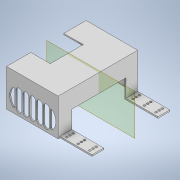
# Autodesk Inventor part: Enclosure
Saved by Autodesk Inventor 2020 (Build 240168000, 168)
## iProperties
Created: 2020-02-08
Part Number: Enclosure
Material: Generic
Document SubType Name: Modeling
Designer: pp445
Density: 1 g/cm^3
Appearance: Default
Author: pp445
Autodesk Inventor part; units mm, degrees
ref_plane "YZ Plane" through (0, 0, 0) normal (1, 0, 0) x (0, 1, 0)
ref_plane "XZ Plane" through (0, 0, 0) normal (0, 1, 0) x (-1, 0, 0)
ref_plane "XY Plane" through (0, 0, 0) normal (0, 0, 1) x (1, 0, 0)
sketch "Sketch1" plane through (0, 0, 0) normal (0, 1, 0) x (-1, 0, 0)
  line L0 (0, 0) -> (81, 0)
  line L1 (81, 0) -> (81, -120)
  line L2 (81, -120) -> (0, -120)
  line L3 (0, -120) -> (0, 0)
  line L4 (217, 30) -> (81, 30)
  line L5 (81, 30) -> (81, -146)
  line L6 (81, -146) -> (217, -146)
  line L7 (217, -146) -> (217, 30)
  line L8 (81, -60) -> (0, -60) construction
  dimension "d0" = 120
  dimension "d1" = 81
  dimension "d2" = 176
  dimension "d4" = 136
  dimension "d40" = 26
  constraints: 18 end point, 4 parallel, 2 horizontal, 2 perpendicular, 1 collinear, 1 midpoint, 1 point on line
  measures "d0" distance of L2.end L0.start
  measures "d1" distance of L0.start L0.end
  measures "d2" distance between parallel lines of L6 L4
  measures "d4" distance of L4.start L4.end
  measures "d40" distance between parallel lines of L2 L6
extrude "Extrusion1" add sketch "Sketch1" against normal blind 82
shell "Shell1" thickness 2.54 removed faces 3 at (-171.6667, -82, -38.6667) at (0, -54.6667, -40) at (-217, -27.3333, -87.3333)
sketch "Sketch3" plane through (0, -82, 0) normal (0, -1, 0) x (1, 0, 0)
  line L0 (-81, -146) -> (-81, -120) projected
  line L1 (0, -2.54) -> (0, 0) projected
  line L2 (0, 0) -> (-81, 0)
  line L3 (-81, -120) -> (0, -120) projected
  line L4 (0, -120) -> (-81, -120)
  line L5 (-81, -120) -> (-81, -146)
  line L6 (-81, -146) -> (0, -146)
  line L7 (0, -146) -> (0, -120)
  line L8 (-81, 0) -> (-81, 30) projected
  line L9 (-81, 0) -> (0, 0) projected
  line L10 (-217, 30) -> (-81, 30) projected
  line L11 (0, 0) -> (-81, 0)
  line L12 (-81, 0) -> (-81, 30)
  line L13 (-81, 30) -> (0, 30)
  line L14 (0, 30) -> (0, 0)
  constraints: 18 end point, 4 parallel, 3 horizontal, 2 perpendicular
extrude "Extrusion3" add sketch "Sketch3" against normal blind 3.175
sketch "Sketch5" plane through (0, -78.825, 0) normal (0, 1, 0) x (1, 0, 0)
  line L0 (0, 120) -> (0, 146) projected
  line L1 (0, 146) -> (-81, 146) projected
  line L2 (-81, 120) -> (-81, 146) projected
  line L3 (0, 120) -> (-81, 120) projected
  line L4 (-81, 0) -> (0, 0) projected
  line L5 (-81, -30) -> (-81, 0) projected
  line L6 (-81, -30) -> (0, -30) projected
  line L7 (0, -30) -> (0, 0) projected
  line L8 (0, 146) -> (0, 117.46) projected
  line L9 (-81, 120) -> (-81, 146) projected
  line L10 (0, 2.54) -> (0, -30) projected
  line L11 (0, -15) -> (-81, -15) construction
  line L12 (-81, -30) -> (-81, 0) projected
  circle A0 centre (-20.7, -15) radius 2.3813
  circle A1 centre (-46.1, -15) radius 2.3813
  circle A2 centre (-71.5, -15) radius 2.3813
  circle A3 centre (-20.7, 133.3) radius 2.3813
  circle A4 centre (-46.1, 133.3) radius 2.3813
  circle A5 centre (-71.5, 133.3) radius 2.3813
  line L13 (-81, 133.3) -> (0, 133.3) construction
  dimension "d18" = 20.7
  dimension "d19" = 25.4
  dimension "d20" = 25.4
  dimension "d21" = 4.7625
  dimension "d22" = 4.7625
  dimension "d23" = 4.7625
  dimension "d41" = 4.7625
  dimension "d42" = 4.7625
  dimension "d43" = 4.7625
  dimension "d44" = 20.7
  dimension "d45" = 25.4
  dimension "d46" = 25.4
  dimension "d47" = 13.3
  constraints: 9 point on line, 6 centre point, 4 end point, 1 midpoint, 1 perpendicular
  measures "d18" distance from line of L7 A0.centre
  measures "d19" distance of A0.centre A1.centre
  measures "d20" distance of A1.centre A2.centre
  measures "d21" diameter of A0
  measures "d22" diameter of A1
  measures "d23" diameter of A2
  measures "d41" diameter of A3
  measures "d42" diameter of A4
  measures "d43" diameter of A5
  measures "d44" distance from line of L8 A3.centre
  measures "d45" distance of A3.centre A4.centre
  measures "d46" distance of A4.centre A5.centre
  measures "d47" distance between parallel lines of L3 L13
extrude "Extrusion4" cut sketch "Sketch5" against normal up to surface (3.175 mm away) contours A3 | A4 | A5
ref_plane "Work Plane1" through (0, -2.54, -60) normal (0, 0, -1) x (-1, 0, 0)
mirror "Mirror1" about plane through (0, -2.54, -60) normal (0, 0, -1) of "Extrusion4"
sketch "Sketch6" plane through (0, 0, 0) normal (0, 1, 0) x (1, 0, 0)
  line L0 (-81, 120) -> (-81, 146) projected
  line L1 (-81, 146) -> (-217, 146) projected
  line L2 (-217, 146) -> (-217, -30) projected
  line L3 (-217, -30) -> (-81, -30) projected
  line L4 (-81, -30) -> (-81, 0) projected
  line L5 (-81, 0) -> (0, 0) projected
  line L6 (0, 0) -> (0, 120) projected
  line L7 (0, 120) -> (-81, 120) projected
  line L8 (-217, 143.46) -> (-217, -27.46) projected
  line L9 (-217, 60) -> (0, 60) construction
  line L10 (-217, 23.5) -> (-152, 23.5)
  line L11 (-152, 23.5) -> (-152, 96.5)
  line L12 (-152, 96.5) -> (-217, 96.5)
  line L13 (-217, 96.5) -> (-217, 23.5)
  line L14 (-217, 60) -> (-152, 60) construction
  dimension "d27" = 65
  constraints: 12 end point, 3 midpoint, 2 parallel, 2 point on line, 1 collinear, 1 horizontal, 1 perpendicular
  measures "d27" distance of L11.end L12.end
extrude "Extrusion5" cut sketch "Sketch6" against normal up to surface (2.54 mm away) contours L12 L11 L10 L2
sketch "Sketch7" plane through (-217, -82, -146) normal (-1, 0, 0) x (0, 0, 1)
  line L0 (0, 82) -> (49.5, 82) projected
  line L1 (49.5, 79.46) -> (49.5, 82) projected
  line L2 (0, 82) -> (49.5, 82) projected
  line L3 (0, 82) -> (0, 0) projected
  line L4 (2.54, 0) -> (0, 0) projected
  line L5 (2.54, 0) -> (2.54, 79.46) projected
  line L6 (2.54, 79.46) -> (49.5, 79.46) projected
  line L7 (122.5, 82) -> (122.5, 79.46) projected
  line L8 (122.5, 79.46) -> (173.46, 79.46) projected
  line L9 (173.46, 79.46) -> (173.46, 0) projected
  line L10 (176, 0) -> (173.46, 0) projected
  line L11 (176, 82) -> (176, 0) projected
  line L12 (122.5, 82) -> (176, 82) projected
  point P0 (146, 82)
  point P1 (49.5, 82)
extrude "Extrusion6" cut sketch "Sketch7" against normal blind 22
mirror "Mirror2" about plane through (0, -2.54, -60) normal (0, 0, -1) of "Extrusion4"
sketch "Sketch9" plane through (0, 0, 0) normal (1, 0, 0) x (0, 0, -1)
  line L0 (2.54, -82) -> (2.54, -2.54) projected
  line L1 (2.54, -2.54) -> (117.46, -2.54) projected
  line L2 (117.46, -2.54) -> (117.46, -82) projected
  line L3 (146, -82) -> (117.46, -82) projected
  line L4 (146, -82) -> (146, -78.825) projected
  line L5 (120, -78.825) -> (146, -78.825) projected
  line L6 (120, 0) -> (120, -78.825) projected
  line L7 (0, 0) -> (120, 0) projected
  line L8 (0, 0) -> (0, -78.825) projected
  line L9 (-30, -78.825) -> (0, -78.825) projected
  line L10 (-30, -82) -> (-30, -78.825) projected
  line L11 (2.54, -82) -> (-30, -82) projected
extrude "Extrusion8" cut sketch "Sketch9" against normal blind 10
sketch "Sketch10" plane through (-10, 0, 0) normal (1, 0, 0) x (0, 0, -1)
  line L0 (2.54, -82) -> (-30, -82) projected
  line L1 (2.54, -2.54) -> (2.54, -82) projected
  line L2 (117.46, -2.54) -> (2.54, -2.54) projected
  line L3 (117.46, -82) -> (117.46, -2.54) projected
  line L4 (146, -82) -> (117.46, -82) projected
  line L5 (146, -78.825) -> (146, -82) projected
  line L6 (120, -78.825) -> (146, -78.825) projected
  line L7 (120, 0) -> (120, -78.825) projected
  line L8 (0, 0) -> (120, 0) projected
  line L9 (0, -78.825) -> (0, 0) projected
  line L10 (-30, -78.825) -> (0, -78.825) projected
  line L11 (-30, -82) -> (-30, -78.825) projected
  line L12 (2.54, -82) -> (-30, -82) projected
  line L13 (-30, -78.825) -> (-26, -78.825)
  line L14 (-26, -78.825) -> (-26, -82)
  line L15 (-26, -82) -> (-30, -82)
  line L16 (-30, -82) -> (-30, -78.825)
  dimension "d50" = 4
  constraints: 8 end point, 2 parallel, 1 horizontal, 1 perpendicular, 1 point on line
  measures "d50" distance between parallel lines of L11 L14
extrude "Extrusion9" cut sketch "Sketch10" against normal up to surface (71 mm away) contours L0 L11 L10 L14
pattern_linear "Rectangular Pattern2" count 2 spacing 7 along (0, 0, -1) count 2 spacing 7 along (0, 0, 1) of "Extrusion4"
mirror "Mirror3" about plane through (0, -2.54, -60) normal (0, 0, -1) of "Extrusion4", "Rectangular Pattern2"
sketch "Sketch11" plane through (-81, -82, 30) normal (0, 0, 1) x (1, 0, 0)
  line L0 (0, 82) -> (0, 0) projected
  line L1 (-114, 82) -> (0, 82) projected
  line L2 (-114, 82) -> (-114, 0) projected
  line L3 (0, 0) -> (-114, 0) projected
  line L4 (-2.54, 0) -> (-114, 0) projected
  line L5 (-3.175, 0) -> (-109.175, 0)
  line L6 (-109.175, 0) -> (-109.175, 58.175)
  line L7 (-109.175, 58.175) -> (-3.175, 58.175)
  line L8 (-3.175, 58.175) -> (-3.175, 0)
  line L9 (-95.5478, 52.5) -> (-95.5478, 7.5)
  circle A0 centre (-79.7364, 30) radius 27.5 construction
  arc A1 (-95.5478, 52.5) -> (-95.5478, 7.5) centre (-79.7364, 30) ccw
  line L10 (-56.175, 58.175) -> (-56.175, 0) construction
  line L11 (-16.8022, 52.5) -> (-16.8022, 7.5)
  circle A2 centre (-32.6136, 30) radius 27.5 construction
  arc A3 (-16.8022, 7.5) -> (-16.8022, 52.5) centre (-32.6136, 30) ccw
  line L12 (-79.7364, 30) -> (-32.6136, 30) construction
  line L13 (-93.0078, 54) -> (-80.3078, 54)
  line L14 (-80.3078, 54) -> (-80.3078, 6)
  line L15 (-80.3078, 6) -> (-93.0078, 6)
  line L16 (-93.0078, 6) -> (-93.0078, 54)
  line L17 (-93.0078, 30) -> (-80.3078, 30) construction
  line L18 (-77.7678, 54) -> (-65.0678, 54)
  line L19 (-65.0678, 54) -> (-65.0678, 6)
  line L20 (-65.0678, 6) -> (-77.7678, 6)
  line L21 (-77.7678, 6) -> (-77.7678, 54)
  line L22 (-62.5278, 54) -> (-49.8278, 54)
  line L23 (-49.8278, 54) -> (-49.8278, 6)
  line L24 (-49.8278, 6) -> (-62.5278, 6)
  line L25 (-62.5278, 6) -> (-62.5278, 54)
  line L26 (-47.2878, 54) -> (-34.5878, 54)
  line L27 (-34.5878, 54) -> (-34.5878, 6)
  line L28 (-34.5878, 6) -> (-47.2878, 6)
  line L29 (-47.2878, 6) -> (-47.2878, 54)
  line L30 (-32.0478, 54) -> (-19.3478, 54)
  line L31 (-19.3478, 54) -> (-19.3478, 6)
  line L32 (-19.3478, 6) -> (-32.0478, 6)
  line L33 (-32.0478, 6) -> (-32.0478, 54)
  point P0 (81, 82)
  point P1 (-65.0678, 30)
  point P2 (-77.7678, 30)
  point P3 (-49.8278, 30)
  point P4 (-62.5278, 30)
  point P5 (-34.5878, 30)
  point P6 (-47.2878, 30)
  point P7 (-19.3478, 30)
  point P8 (-32.0478, 30)
  dimension "d59" = 3.175
  dimension "d60" = 106
  dimension "d61" = 58.175
  dimension "d62" = 45
  dimension "d63" = 55
  dimension "d64" = 30
  dimension "d66" = 29.4386
  dimension "d70" = 48
  dimension "d71" = 2.54
  dimension "d72" = 12.7
  dimension "d83" = 15.24
  constraints: 58 end point, 8 point on circle, 4 centre point, 4 horizontal, 4 midpoint, 4 parallel, 4 symmetric about line, 3 perpendicular, 2 coincident, 1 collinear, 1 point on line, 1 vertical, 42 other
  measures "d59" distance between parallel lines of L0 L8
  measures "d60" distance of L6.end L7.end
  measures "d61" distance of L5.end L6.end
  measures "d62" distance of L9.start L9.end
  measures "d63" diameter of A0
  measures "d64" distance from line of L3 A0.centre
  measures "d66" distance from line of L6 A0.centre
  measures "d70" distance of L13.end L14.end
  measures "d71" distance between parallel lines of L9 L16
  measures "d72" distance between parallel lines of L16 L14
  measures "d83" distance of L13.start L18.start
extrude "Extrusion10" cut sketch "Sketch11" against normal up to surface (2.54 mm away) contours L9 A1 | A3 L11 | L13 L14 L15 L16 | L18 L19 L20 L21 | L22 L23 L24 L25 | L26 L27 L28 L29 | L30 L31 L32 L33
fillet "Fillet1" radius 2.54 4 edges at (-176.5478, -29.5, 28.73) (-176.5478, -74.5, 28.73) (-97.8022, -29.5, 28.73) (-97.8022, -74.5, 28.73)
fillet "Fillet2" radius 6.35 20 edges at (-174.0078, -76, 28.73) (-161.3078, -76, 28.73) (-161.3078, -28, 28.73) (-174.0078, -28, 28.73) (-158.7678, -76, 28.73) (-143.5278, -76, 28.73) (-128.2878, -76, 28.73) (-113.0478, -76, 28.73) (-100.3478, -76, 28.73) (-115.5878, -76, 28.73) (-130.8278, -76, 28.73) (-146.0678, -76, 28.73) (-158.7678, -28, 28.73) (-143.5278, -28, 28.73) (-128.2878, -28, 28.73) (-113.0478, -28, 28.73) (-100.3478, -28, 28.73) (-115.5878, -28, 28.73) (-130.8278, -28, 28.73) (-146.0678, -28, 28.73)
sketch "Sketch12" plane through (-10, 0, 0) normal (1, 0, 0) x (0, 0, -1)
  line L0 (-26, -78.825) -> (-26, -82) projected
  line L1 (2.54, -82) -> (-26, -82) projected
  line L2 (2.54, -2.54) -> (2.54, -82) projected
  line L3 (117.46, -2.54) -> (2.54, -2.54) projected
  line L4 (117.46, -82) -> (117.46, -2.54) projected
  line L5 (146, -82) -> (117.46, -82) projected
  line L6 (146, -78.825) -> (146, -82) projected
  line L7 (120, -78.825) -> (146, -78.825) projected
  line L8 (120, 0) -> (120, -78.825) projected
  line L9 (0, 0) -> (120, 0) projected
  line L10 (0, -78.825) -> (0, 0) projected
  line L11 (-26, -78.825) -> (0, -78.825) projected
  line L12 (0, -78.825) -> (0, 0) projected
  line L13 (2.54, -82) -> (0, -82)
  line L14 (0, -82) -> (0, 0)
  line L15 (0, 0) -> (2.54, 0)
  line L16 (2.54, 0) -> (2.54, -82)
  line L17 (117.46, -82) -> (143.46, -82) projected
  line L18 (120, 0) -> (120, -78.825) projected
  line L19 (117.46, -82) -> (120, -82)
  line L20 (120, -82) -> (120, 0)
  line L21 (120, 0) -> (117.46, 0)
  line L22 (117.46, 0) -> (117.46, -82)
  line L23 (117.46, 0) -> (2.54, 0)
  line L24 (2.54, 0) -> (2.54, -2.54)
  line L25 (2.54, -2.54) -> (117.46, -2.54)
  line L26 (117.46, -2.54) -> (117.46, 0)
  constraints: 24 end point, 6 parallel, 3 horizontal, 3 perpendicular
extrude "Extrusion11" cut sketch "Sketch12" against normal up to surface (73.54 mm away) contours L10 L9 L16 L2 L1 L14 | L9 L22 L3 L16 | L9 L8 L20 L5 L4 L22
sketch "Sketch13" plane through (-83.54, -2.54, -120) normal (1, 0, 0) x (0, 0, -1)
  line L0 (-120, 2.54) -> (0, 2.54) projected
  line L1 (-120, 0) -> (0, 0) projected
  line L2 (0, 2.54) -> (0, 0) projected
  line L3 (-120, 2.54) -> (0, 2.54) projected
  line L4 (-120, 0) -> (-120, 2.54) projected
  line L5 (0, 2.54) -> (-120, 2.54)
  line L6 (-120, 2.54) -> (-120, -37.46)
  line L7 (-120, -37.46) -> (0, -37.46)
  line L8 (0, -37.46) -> (0, 2.54)
  dimension "d90" = 40
  constraints: 8 end point, 2 parallel, 1 horizontal, 1 perpendicular
  measures "d90" distance between parallel lines of L0 L7
extrude "Extrusion12" add sketch "Sketch13" along normal up to surface (2.54 mm away)
equation "\"d20\" = d19"
equation "\"d22\" = d21"
equation "\"d23\" = d21"
equation "\"d41\" = d21"
equation "\"d42\" = d41"
equation "\"d43\" = d41"
equation "\"d44\" = d18"
equation "\"d45\" = d19"
equation "\"d46\" = d45"
body "Solid1"
